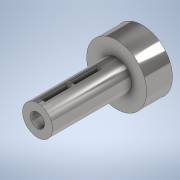
# Autodesk Inventor part: Носок
Saved by Autodesk Inventor 2021 (Build 250183000, 183)
## iProperties
Created: 2020-12-13
Part Number: Носок
Material: Сталь, высокопрочная, низколегированная
Document SubType Name: Modeling
Designer: panda
Mass: 1691.61 g
Surface Area: 275.927 cm^2
Volume: 215.492 cm^3
Density: 7.85 g/cm^3
Appearance: Сталь — полированная
Author: panda
Autodesk Inventor part; units mm, degrees
ref_plane "YZ Plane" through (0, 0, 0) normal (1, 0, 0) x (0, 1, 0)
ref_plane "XZ Plane" through (0, 0, 0) normal (0, 1, 0) x (-1, 0, 0)
ref_plane "XY Plane" through (0, 0, 0) normal (0, 0, 1) x (1, 0, 0)
sketch "Эскиз1" plane through (0, 0, 0) normal (0, 0, 1) x (1, 0, 0)
  circle A0 centre (0, 0) radius 36
  dimension "d0" = 72
  constraints: 1 centre point, 1 coincident
  measures "d0" diameter of A0
extrude "Выдавливание1" add sketch "Эскиз1" along normal blind 31
sketch "Эскиз2" plane through (0, 0, 31) normal (0, 0, 1) x (1, 0, 0)
  circle A0 centre (0, 0) radius 18
  dimension "d3" = 36
  constraints: 1 centre point, 1 coincident
  measures "d3" diameter of A0
extrude "Выдавливание2" add sketch "Эскиз2" along normal blind 95
sketch "Эскиз3" plane through (0, 0, 126) normal (0, 0, 1) x (1, 0, 0)
  point P0 (0, -47.75)
  point P1 (0, 0)
hole "Отверстие1" at (0, 0, 126) direction (0, 0, -1) diameter 17 depth 31 tip angle 118
sketch "Эскиз4" plane through (0, 0, 0) normal (1, 0, 0) x (0, 1, 0)
  line L0 (18, 31) -> (18, 126) projected
  line L1 (18, 120) -> (18, 88)
  line L2 (18, 126) -> (-18, 126) projected
  line L3 (18, 120) -> (11.5, 120)
  line L4 (11.5, 120) -> (11.5, 88)
  line L5 (11.5, 88) -> (18, 88)
  arc A0 (11.5, 120) -> (11.5, 88) centre (48.1606, 104) ccw
  line L6 (18, 84) -> (18, 52)
  line L7 (18, 84) -> (11.5, 84)
  line L8 (11.5, 84) -> (11.5, 52)
  line L9 (11.5, 52) -> (18, 52)
  arc A1 (11.5, 84) -> (11.5, 52) centre (48.1606, 68) ccw
  point P0 (0, 0)
  point P1 (19, 127)
  dimension "d13" = 6
  dimension "d14" = 32
  dimension "d15" = 6.5
  dimension "d16" = 40
  dimension "d17" = 32
  dimension "d18" = 6.5
  dimension "d19" = 40
  dimension "d20" = 4
  constraints: 16 end point, 6 perpendicular, 4 point on circle, 3 point on line, 2 centre point
  measures "d13" distance from line of L2 L1.start
  measures "d14" distance of L1.start L1.end
  measures "d15" distance of L1.start L3.end
  measures "d16" radius of A0
  measures "d17" distance of L6.start L6.end
  measures "d18" distance of L6.start L7.end
  measures "d19" radius of A1
  measures "d20" distance of L1.end L6.start
extrude "Выдавливание3" cut sketch "Эскиз4" against normal mid plane 6
